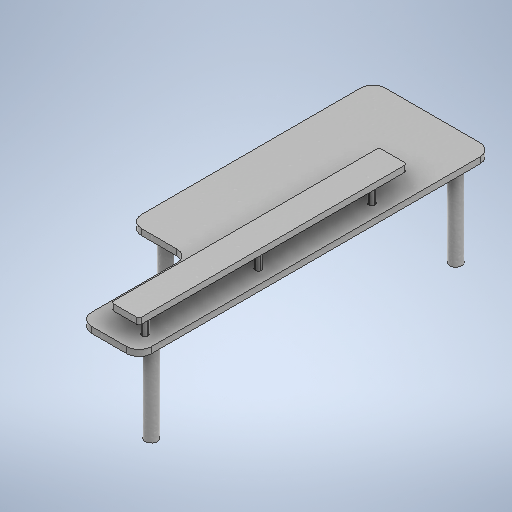
# Autodesk Inventor part: mesa_001
Saved by Autodesk Inventor 2026 (Build 300175000, 175)
## iProperties
Created: 2025-05-30
Part Number: mesa_001
Material: ABS Plastic
Document SubType Name: Modeling
Designer: Carlos Dias
Density: 1.06 g/cm^3
Appearance: Textured - Gray
Author: Carlos Dias
## iProperties of the stored document mesa_001_3DPrint.ipt
Created: 2025-05-30
Part Number: mesa_001_3DPrint
Material: Generic
Document SubType Name: Modeling
Designer: Carlos Dias
Density: 1 g/cm^3
Appearance: Default
Author: Carlos Dias
Autodesk Inventor part; units mm, degrees
sketch "Sketch1" plane through (0, 0, 0) normal (0, 1, 0) x (-1, 0, 0)
  line L0 (49, -100) -> (-49, -100)
  line L1 (-49, -100) -> (-49, 100)
  line L2 (-49, 100) -> (49, 100)
  line L3 (49, 100) -> (49, -100)
  line L4 (0, 100) -> (-49, 100)
  line L5 (-49, 100) -> (-49, 190)
  line L6 (-49, 190) -> (0, 190)
  line L7 (0, 190) -> (0, 100)
  point P0 (0, 0)
  point P1 (0, -100)
  point P2 (-49, 0)
  dimension "d0" = 98
  dimension "d1" = 200
  dimension "d2" = 90
  constraints: 16 end point, 4 parallel, 2 horizontal, 2 midpoint, 2 perpendicular, 2 vertical alignment, 1 coincident, 1 horizontal alignment, 1 point on line
  measures "d0" distance of L0.start L0.end
  measures "d1" distance of L0.end L1.end
  measures "d2" distance of L4.end L5.end
extrude "Extrusion1" add sketch "Sketch1" along normal mid plane 5
sketch "Sketch2" plane through (0, -2.5, 0) normal (0, -1, 0) x (1, 0, 0)
  line L0 (-39, -90) -> (-29, -90)
  line L1 (-29, -90) -> (-29, -80)
  line L2 (-29, -80) -> (-39, -80)
  line L3 (-39, -80) -> (-39, -90)
  line L4 (29, -90) -> (39, -90)
  line L5 (39, -90) -> (39, -80)
  line L6 (39, -80) -> (29, -80)
  line L7 (29, -80) -> (29, -90)
  line L8 (-39, 80) -> (-29, 80)
  line L9 (-29, 80) -> (-29, 90)
  line L10 (-29, 90) -> (-39, 90)
  line L11 (-39, 90) -> (-39, 80)
  line L12 (29, 160) -> (39, 160)
  line L13 (39, 160) -> (39, 170)
  line L14 (39, 170) -> (29, 170)
  line L15 (29, 170) -> (29, 160)
  point P0 (0, 0)
  dimension "d5" = 10
  dimension "d6" = 80
  dimension "d7" = 29
  dimension "d8" = 29
  dimension "d9" = 80
  dimension "d10" = 80
  dimension "d11" = 29
  dimension "d12" = 29
  dimension "d14" = 170
  constraints: 32 end point, 8 parallel, 7 equal length, 4 horizontal, 4 perpendicular
  measures "d5" distance of L2.end L0.start
  measures "d6" distance from line of point (0, 0) L2
  measures "d7" distance from line of point (0, 0) L1
  measures "d8" distance from line of point (0, 0) L7
  measures "d9" distance from line of point (0, 0) L6
  measures "d10" distance from line of point (0, 0) L8
  measures "d11" distance from line of point (0, 0) L9
  measures "d12" distance from line of L15 point (0, 0)
  measures "d14" distance from line of point (0, 0) L14
extrude "Extrusion2" add sketch "Sketch2" along normal blind 75
sketch "Sketch3" plane through (0, 2.5, 0) normal (0, 1, 0) x (1, 0, 0)
  line L0 (35, 15) -> (40, 15)
  line L1 (40, 15) -> (40, 10)
  line L2 (40, 10) -> (35, 10)
  line L3 (35, 10) -> (35, 15)
  line L4 (35, -78) -> (40, -78)
  line L5 (40, -78) -> (40, -83)
  line L6 (40, -83) -> (35, -83)
  line L7 (35, -83) -> (35, -78)
  line L8 (35, -171) -> (40, -171)
  line L9 (40, -171) -> (40, -176)
  line L10 (40, -176) -> (35, -176)
  line L11 (35, -176) -> (35, -171)
  point P0 (0, 0)
  point P1 (37.5, 15)
  point P2 (37.5, -78)
  point P3 (37.5, 10)
  point P4 (37.5, -171)
  point P5 (37.5, -83)
  point P6 (37.5, -176)
  dimension "d21" = 88
  dimension "d22" = 88
  dimension "d30" = 35
  dimension "d31" = 10
  dimension "d32" = 5
  constraints: 24 end point, 6 midpoint, 6 parallel, 5 equal length, 3 horizontal, 3 perpendicular, 2 vertical alignment
  measures "d21" distance between parallel lines of L4 L2
  measures "d22" distance between parallel lines of L8 L6
  measures "d30" distance from line of point (0, 0) L3
  measures "d31" distance from line of point (0, 0) L2
  measures "d32" distance of L0.end L1.end
extrude "Extrusion3" add sketch "Sketch3" along normal blind 20
sketch "Sketch4" plane through (0, 22.5, 0) normal (0, 1, 0) x (1, 0, 0)
  line L0 (26, 30) -> (49, 30)
  line L1 (49, 30) -> (49, -190)
  line L2 (49, -190) -> (26, -190)
  line L3 (26, -190) -> (26, 30)
  point P0 (0, 0)
  point P1 (37.5, 30)
  point P2 (49, 100)
  point P3 (37.5, -190)
  point P4 (49, -80)
  dimension "d33" = 220
  dimension "d34" = 23
  constraints: 8 end point, 3 horizontal alignment, 3 midpoint, 2 parallel, 2 vertical alignment
  measures "d33" distance of L0.end L1.end
  measures "d34" distance of L0.start L0.end
extrude "Extrusion4" add sketch "Sketch4" along normal blind 5
fillet "Fillet1" radius 10 6 edges at (-49, 0, -100) (49, 0, -100) (-49, 0, 100) (0, 0, 100) (0, 0, 190) (49, 0, 190)
fillet "Fillet2" radius 2 16 edges at (26, 25, 190) (49, 25, 190) (26, 25, -30) (49, 25, -30) (35, 12.5, -10) (35, 12.5, -15) (40, 12.5, -10) (40, 12.5, -15) (35, 12.5, 78) (35, 12.5, 83) (40, 12.5, 83) (40, 12.5, 78) (35, 12.5, 176) (35, 12.5, 171) (40, 12.5, 176) (40, 12.5, 171)
fillet "Fillet3" radius 5 16 edges at (-39, -40, 90) (-39, -40, 80) (-29, -40, 90) (-29, -40, 80) (29, -40, 170) (29, -40, 160) (39, -40, 160) (39, -40, 170) (-39, -40, -80) (-39, -40, -90) (-29, -40, -90) (-29, -40, -80) (29, -40, -80) (29, -40, -90) (39, -40, -90) (39, -40, -80)
equation "\"d8\" = d7"
equation "\"d9\" = d6"
equation "\"d10\" = d6"
equation "\"d11\" = d7"
equation "\"d12\" = d7"
equation "\"d21\" = d20"
equation "\"d22\" = d20"
equation "\"d20\" = 88"
body "Solid1"
